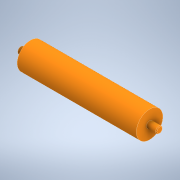
# Autodesk Inventor part: Roller Pin
Saved by Autodesk Inventor 2022.4 (Build 264492000, 492)
## iProperties
Created: 2024-02-15
Part Number: Roller Pin
Material: Generic
Document SubType Name: Modeling
Designer: t60147996
Density: 1 g/cm^3
Appearance: Orange
Author: t60147996
Autodesk Inventor part; units mm, degrees
ref_plane "YZ Plane" through (0, 0, 0) normal (1, 0, 0) x (0, 1, 0)
ref_plane "XZ Plane" through (0, 0, 0) normal (0, 1, 0) x (-1, 0, 0)
ref_plane "XY Plane" through (0, 0, 0) normal (0, 0, 1) x (1, 0, 0)
sketch "Sketch1" plane through (0, 0, 0) normal (1, 0, 0) x (0, 1, 0)
  circle A0 centre (0, 0) radius 25.4
  dimension "d0" = 50.8
  constraints: 1 centre point, 1 coincident
  measures "d0" diameter of A0
extrude "Extrusion1" add sketch "Sketch1" along normal blind 228.6
sketch "Sketch2" plane through (228.6, 0, 0) normal (1, 0, 0) x (0, 0, -1)
  circle A0 centre (0, 0) radius 6.35
  dimension "d3" = 12.7
  constraints: 2 coincident, 1 centre point
  measures "d3" diameter of A0
extrude "Extrusion2" add sketch "Sketch2" along normal blind 19.05
chamfer "Chamfer1" distance 1.27 angle 45 1 edges at (247.65, 0, 6.35)
sketch "Sketch3" plane through (0, 0, 0) normal (-1, 0, 0) x (0, 0, 1)
  circle A0 centre (0, 0) radius 6.35 projected
  circle A1 centre (0, 0) radius 6.35
  constraints: 1 centre point, 1 coincident
extrude "Extrusion3" add sketch "Sketch3" along normal blind 19.05
chamfer "Chamfer2" distance 1.27 angle 45 1 edges at (-19.05, 0, -6.35)
body "Solid1"
